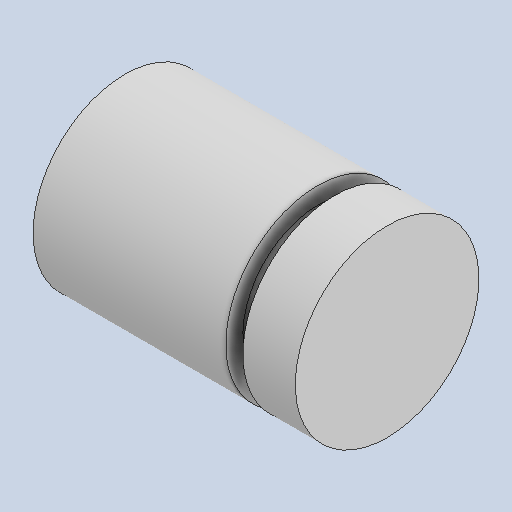
# Autodesk Inventor part: MainAxis_GC_Feder_Fixation_CapstonDisc
Saved by Autodesk Inventor 2022 (Build 260153000, 153)
## iProperties
Created: 2022-07-25
Part Number: MainAxis_GC_Feder_Fixation_CapstonDisc
Material: Generisch
Document SubType Name: Modeling
Designer: alexw
Density: 1 g/cm^3
Appearance: Vorgabe
Mass: 2.87155 g
Surface Area: 14.1275 cm^2
Volume: 2.87155 cm^3
Author: alexw
Autodesk Inventor part; units mm, degrees
ref_plane "YZ Plane" through (0, 0, 0) normal (1, 0, 0) x (0, 1, 0)
ref_plane "XZ Plane" through (0, 0, 0) normal (0, 1, 0) x (-1, 0, 0)
ref_plane "XY Plane" through (0, 0, 0) normal (0, 0, 1) x (1, 0, 0)
sketch "Skizze1" plane through (0, 0, 0) normal (0, 0, 1) x (1, 0, 0)
  line L0 (0, 0) -> (0, 7)
  line L1 (0, 7) -> (14.7, 7)
  line L2 (14.7, 7) -> (14.7, 5.7)
  line L3 (14.7, 5.7) -> (16, 5.7)
  line L4 (16, 5.7) -> (16, 7)
  line L5 (16, 7) -> (20, 7)
  line L6 (20, 7) -> (20, 0)
  line L7 (20, 0) -> (0, 0)
  dimension "d0" = 14
  dimension "d1" = 20
  dimension "d2" = 4
  dimension "d3" = 1.3
  dimension "d4" = 1.3
  constraints: 16 end point, 6 perpendicular, 2 point on line, 1 vertical
  measures "d0" diameter of L1 L7
  measures "d1" distance between parallel lines of L0 L6
  measures "d2" distance between parallel lines of L6 L4
  measures "d3" distance of L2.end L3.end
  measures "d4" distance between parallel lines of L1 L3
revolve "Umdrehung1" add sketch "Skizze1" angle 360 about axis through (20, 0, 0) along (-1, 0, 0)
sketch "Skizze2" plane through (0, 0, 0) normal (-1, 0, 0) x (0, 0, 1)
  point P0 (0, 0)
  point P1 (0, 0)
  constraints: 1 coincident
hole "Bohrung1" at (0, 0, 0) direction (1, 0, 0) diameter 4.134 depth 10 tip angle 118 thread size "M5x0.8" class "6H" standard "ISO Metric profile"
